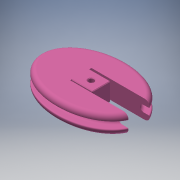
# Autodesk Inventor part: climb pulley
Saved by Autodesk Inventor 2017 SP1 (Build 210196100, 196)
## iProperties
Created: 2018-03-22
Part Number: climb pulley
Material: Generic
Document SubType Name: Modeling
Designer: Ben
Density: 1 g/cm^3
Appearance: Pink
Author: Ben
Autodesk Inventor part; units mm, degrees
ref_plane "YZ Plane" through (0, 0, 0) normal (1, 0, 0) x (0, 1, 0)
ref_plane "XZ Plane" through (0, 0, 0) normal (0, 1, 0) x (-1, 0, 0)
ref_plane "XY Plane" through (0, 0, 0) normal (0, 0, 1) x (1, 0, 0)
sketch "Sketch1" plane through (0, 0, 0) normal (0, 0, 1) x (1, 0, 0)
  line L0 (38.1, 11.1125) -> (38.1, -11.1125)
  line L1 (0, 0) -> (38.1, 0) construction
  arc A0 (54.7687, 3.9688) -> (54.7687, -3.9688) centre (54.7687, 0) ccw
  line L2 (54.7687, 3.9688) -> (59.8487, 3.9688)
  line L3 (54.7687, -3.9688) -> (59.8487, -3.9688)
  line L4 (61.1187, 5.2387) -> (61.1187, 5.5245)
  line L5 (61.1187, -5.2387) -> (61.1187, -5.5245)
  arc A1 (61.1187, 5.5245) -> (55.5307, 11.1125) centre (55.5307, 5.5245) ccw
  line L6 (55.5307, 11.1125) -> (38.1, 11.1125)
  line L7 (38.1, -11.1125) -> (55.5307, -11.1125)
  arc A2 (55.5307, -11.1125) -> (61.1187, -5.5245) centre (55.5307, -5.5245) ccw
  arc A3 (59.8487, 3.9688) -> (61.1187, 5.2387) centre (59.8487, 5.2387) ccw
  arc A4 (61.1187, -5.2387) -> (59.8487, -3.9688) centre (59.8487, -5.2387) ccw
  point P0 (61.1187, 3.9688)
  point P1 (50.8, 0)
  dimension "d1" = 22.225
  dimension "d5" = 6.35
  dimension "d6" = 7.9375
  dimension "d7" = 1.27
  dimension "d8" = 5.588
  dimension "d30" = 12.7
  dimension "d31" = 50.8
  constraints: 16 end point, 11 point on circle, 10 tangent, 5 centre point, 4 horizontal, 3 point on line, 3 vertical, 2 coincident, 2 equal length, 2 equal radius, 1 midpoint
  measures "d1" distance of L0.start L0.end
  measures "d5" distance of L2.start point (61.119, 3.969)
  measures "d6" diameter of A0
  measures "d7" radius of A3
  measures "d8" radius of A1
  measures "d30" distance from line of L0 point (50.8, 0)
  measures "d31" distance of point (0, 0) point (50.8, 0)
sketch "Sketch2" plane through (0, 0, 0) normal (0, 1, 0) x (-1, 0, 0)
  ellipse E0 centre (0, 0) end of major axis (-50.8, 0) minor radius 31.75
  dimension "d9" = 50.8
  dimension "d10" = 31.75
  constraints: 1 coincident, 2 other
sweep "Sweep1" add profiles "Sketch1" path "Sketch2"
sketch "Sketch3" plane through (0, 0, 0) normal (0, 1, 0) x (-1, 0, 0)
  spline S0 degree 5 poles (-38.1, 0) (-38.1008, -1.0764) (-37.8929, -2.1558) (-37.4997, -3.172) (-36.5006, -5.0897) (-35.1524, -6.7819) (-34.4217, -7.5754) (-32.8648, -9.0681) (-31.1586, -10.3859) (-30.2759, -11.0051) (-28.4631, -12.1697) (-26.5685, -13.1966) (-25.6045, -13.6777) (-23.6479, -14.5795) (-21.6422, -15.3658) (-20.629, -15.7316) (-18.5849, -16.4106) (-16.5098, -16.9883) (-15.4658, -17.2527) (-13.3665, -17.7341) (-11.2482, -18.123) (-10.185, -18.295) (-8.0523, -18.5946) (-5.9091, -18.8071) (-4.8356, -18.8918) (-2.6857, -19.0186) (-0.5324, -19.0606) (0.5446, -19.0605) (2.6978, -19.018) (4.8478, -18.8908) (5.9213, -18.8058) (8.0646, -18.5931) (10.1973, -18.2931) (11.2605, -18.1211) (13.3788, -17.7317) (15.4781, -17.2498) (16.522, -16.985) (18.5971, -16.4068) (20.6411, -15.7274) (21.6543, -15.3613) (23.6598, -14.5744) (25.6162, -13.6721) (26.5799, -13.1906) (28.4743, -12.1631) (30.2867, -10.9978) (31.1692, -10.3782) (32.8743, -9.06) (34.4304, -7.5664) (35.1597, -6.7729) (36.5077, -5.0799) (37.5034, -3.1628) (37.8968, -2.1443) (38.3066, 0.0102) (37.8908, 2.1635) (37.4957, 3.1812) (36.4959, 5.0964) (35.1468, 6.7884) (34.4162, 7.581) (32.859, 9.0731) (31.1529, 10.3899) (30.2703, 11.0089) (28.4577, 12.1728) (26.5634, 13.1992) (25.5996, 13.6801) (23.6433, 14.5814) (21.6381, 15.3674) (20.625, 15.733) (18.5813, 16.4116) (16.5067, 16.9891) (15.4629, 17.2533) (13.3641, 17.7346) (11.2463, 18.1233) (10.1834, 18.2952) (8.0512, 18.5948) (5.9085, 18.8071) (4.8352, 18.8918) (2.6858, 19.0186) (0.5331, 19.0606) (-0.5436, 19.0605) (-2.6964, 19.0181) (-4.8459, 18.8909) (-5.9192, 18.806) (-8.0619, 18.5934) (-10.1941, 18.2936) (-11.2571, 18.1217) (-13.3749, 17.7325) (-15.4737, 17.2509) (-16.5175, 16.9862) (-18.592, 16.4084) (-20.6357, 15.7293) (-21.6486, 15.3635) (-23.6537, 14.577) (-25.6098, 13.6752) (-26.5734, 13.194) (-28.4675, 12.1671) (-30.2798, 11.0025) (-31.1622, 10.3834) (-32.8675, 9.0657) (-34.4236, 7.5735) (-35.1534, 6.7801) (-36.5015, 5.0888) (-37.4999, 3.1715) (-37.8924, 2.1553) (-38.1013, 1.0763) (-38.1, 0) knots 0 0 0 0 0 0 0.029412 0.029412 0.029412 0.058825 0.058825 0.058825 0.088242 0.088242 0.088242 0.11766 0.11766 0.11766 0.147079 0.147079 0.147079 0.176494 0.176494 0.176494 0.20591 0.20591 0.20591 0.235325 0.235325 0.235325 0.264742 0.264742 0.264742 0.294157 0.294157 0.294157 0.323575 0.323575 0.323575 0.352991 0.352991 0.352991 0.38241 0.38241 0.38241 0.411828 0.411828 0.411828 0.441246 0.441246 0.441246 0.470649 0.470649 0.470649 0.500054 0.500054 0.500054 0.52946 0.52946 0.52946 0.558866 0.558866 0.558866 0.588276 0.588276 0.588276 0.617687 0.617687 0.617687 0.647099 0.647099 0.647099 0.676507 0.676507 0.676507 0.705916 0.705916 0.705916 0.735324 0.735324 0.735324 0.764734 0.764734 0.764734 0.794143 0.794143 0.794143 0.823553 0.823553 0.823553 0.852962 0.852962 0.852962 0.882374 0.882374 0.882374 0.911786 0.911786 0.911786 0.941196 0.941196 0.941196 0.970592 0.970592 0.970592 1 1 1 1 1 1 projected
  circle A0 centre (0, 0) radius 3.302
  dimension "d23" = 6.604
  constraints: 1 centre point, 1 coincident, 1 other
  measures "d23" diameter of A0
extrude "Extrusion1" add sketch "Sketch3" along normal mid plane 21.971
sketch "Sketch4" plane through (-0.0114, 11.1125, -0.0005) normal (0, 1, 0) x (1, 0, 0)
  circle A0 centre (0.0114, -0.0005) radius 3.302 projected
  line L0 (0.0114, -0.0005) -> (12.7114, -0.0005) construction
  line L1 (12.7114, 10.985) -> (12.7114, -10.986)
  line L2 (12.7114, -10.986) -> (-12.6886, -10.986)
  line L3 (-12.6886, -10.986) -> (-12.6886, -12.9545)
  line L4 (-12.6886, -12.9545) -> (88.9114, -12.9545)
  line L5 (88.9114, -12.9545) -> (88.9114, 12.9535)
  line L6 (88.9114, 12.9535) -> (-12.6886, 12.9535)
  line L7 (-12.6886, 12.9535) -> (-12.6886, 10.985)
  line L8 (-12.6886, 10.985) -> (12.7114, 10.985)
  dimension "d25" = 12.7
  dimension "d26" = 12.7
  dimension "d27" = 21.971
  dimension "d29" = 101.6
  dimension "d32" = 25.908
  constraints: 18 end point, 6 perpendicular, 2 collinear, 2 horizontal, 1 midpoint, 1 vertical, 1 other
  measures "d25" distance from line of L0.start L7
  measures "d26" distance of L0.start L0.end
  measures "d27" distance between parallel lines of L2 L8
  measures "d29" distance of L5.end L6.end
  measures "d32" distance between parallel lines of L4 L6
extrude "Extrusion2" cut sketch "Sketch4" against normal through all contours L8 L7 L6 L5 L4 L3 L2 L1
chamfer "Chamfer1" distance 0.762 angle 45 10 edges at (12.7, 10.9855, 0) (12.7, 0, -10.9855) (0, 10.9855, -10.9855) (0, 10.9855, 10.9855) (12.7, 0, 10.9855) (12.7, -10.9855, 0) (0, -10.9855, 10.9855) (0, -10.9855, -10.9855) (3.302, -10.9855, 0) (3.302, 10.9855, 0)
body "Solid1"
